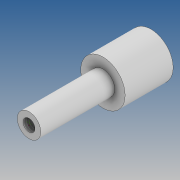
# Autodesk Inventor part: 202.004.01_Zapfen_Aktor
Saved by Autodesk Inventor 2021 (Build 250183000, 183)
## iProperties
Created: 2021-11-26
Part Number: 202.004.01_Zapfen_Aktor
Material: Generisch
Document SubType Name: Modeling
Designer: Oliver Ungerer
Density: 1 g/cm^3
Appearance: Vorgabe
Author: Oliver Ungerer
Autodesk Inventor part; units mm, degrees
ref_plane "YZ Plane" through (0, 0, 0) normal (1, 0, 0) x (0, 1, 0)
ref_plane "XZ Plane" through (0, 0, 0) normal (0, 1, 0) x (-1, 0, 0)
ref_plane "XY Plane" through (0, 0, 0) normal (0, 0, 1) x (1, 0, 0)
sketch "Skizze1" plane through (0, 0, 0) normal (1, 0, 0) x (0, 1, 0)
  line L0 (6, 0) -> (6, 13)
  line L1 (6, 13) -> (3.175, 13)
  line L2 (3.175, 13) -> (3.175, 33)
  line L3 (3.175, 33) -> (0, 33)
  line L4 (0, 33) -> (0, 0)
  line L5 (0, 0) -> (6, 0)
  dimension "d0" = 6
  dimension "d1" = 3.175
  dimension "d2" = 13
  dimension "d3" = 20
  constraints: 12 end point, 5 perpendicular, 1 vertical
  measures "d0" distance between parallel lines of L4 L0
  measures "d1" distance between parallel lines of L4 L2
  measures "d2" distance between parallel lines of L5 L1
  measures "d3" distance between parallel lines of L1 L3
revolve "Umdrehung1" add sketch "Skizze1" angle 360 about axis through (0, 0, 33) along (0, 0, -1)
sketch "Skizze2" plane through (0, 0, 33) normal (0, 0, 1) x (1, 0, 0)
  point P0 (0, 0)
  point P1 (0.0356, 0.5424)
hole "Bohrung1" at (0, 0, 0) direction (0, 0, 1) diameter 3.242 depth 33 tip angle 118 thread size "M4x0.7" class "6H" standard "ISO Metric profile"
